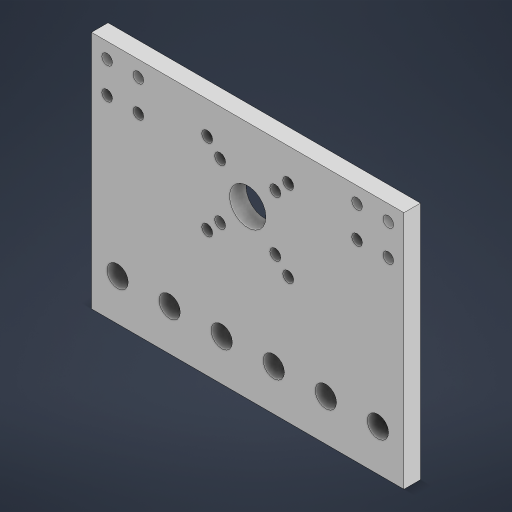
# Autodesk Inventor part: FirstStageMotorMountingPlate
Saved by Autodesk Inventor 2024 (Build 280153000, 153)
## iProperties
Created: 2024-01-05
Part Number: FirstStageMotorMountingPlate
Material: Generic
Document SubType Name: Modeling
Designer: avsar
Density: 1 g/cm^3
Appearance: Default
Author: avsar
Autodesk Inventor part; units mm, degrees
ref_plane "YZ Plane" through (0, 0, 0) normal (1, 0, 0) x (0, 1, 0)
ref_plane "XZ Plane" through (0, 0, 0) normal (0, 1, 0) x (-1, 0, 0)
ref_plane "XY Plane" through (0, 0, 0) normal (0, 0, 1) x (1, 0, 0)
sketch "Sketch1" plane through (0, 0, 0) normal (0, 0, 1) x (1, 0, 0)
  line L0 (-60, -46) -> (60, -46)
  line L1 (60, -46) -> (60, 46)
  line L2 (60, 46) -> (-60, 46)
  line L3 (-60, 46) -> (-60, -46)
  line L4 (-60, -46) -> (60, 46) construction
  line L5 (60, -46) -> (-60, 46) construction
  point P0 (0, 0)
  dimension "d0" = 120
  dimension "d1" = 92
  constraints: 12 end point, 2 midpoint, 2 parallel, 1 horizontal, 1 perpendicular
  measures "d0" distance of L2.end L1.end
  measures "d1" distance of L1.end L0.end
extrude "Extrusion1" add sketch "Sketch1" along normal mid plane 6.35
sketch "Sketch2" plane through (0, 0, 3.175) normal (0, 0, 1) x (1, 0, 0)
  circle A0 centre (0, 18) radius 7
  line L0 (-60, -46) -> (60, -46) projected
  circle A1 centre (-10.6066, 28.6066) radius 2.1
  line L1 (-10.6066, 28.6066) -> (0, 18) construction
  circle A2 centre (-15.5563, 33.5563) radius 2.1
  line L2 (-15.5563, 33.5563) -> (-10.6066, 28.6066) construction
  circle A3 centre (-15.5563, 2.4437) radius 2.1
  circle A4 centre (-10.6066, 7.3934) radius 2.1
  circle A5 centre (15.5563, 2.4437) radius 2.1
  circle A6 centre (10.6066, 7.3934) radius 2.1
  circle A7 centre (15.5563, 33.5563) radius 2.1
  circle A8 centre (10.6066, 28.6066) radius 2.1
  point P0 (0, 0)
  point P1 (0, -46)
  dimension "d4" = 14
  dimension "d6" = 64
  dimension "d7" = 4.2
  dimension "d8" = 45
  dimension "d9" = 15
  dimension "d10" = 4.2
  dimension "d11" = 7
  dimension "d14" = 360
  constraints: 9 centre point, 4 end point, 1 collinear, 1 midpoint, 1 vertical alignment, 17 other
  measures "d4" diameter of A0
  measures "d6" distance of point (0, -46) L1.end
  measures "d7" diameter of A1
  measures "d8" angle of L0 L1
  measures "d9" distance of L1.start L1.end
  measures "d10" diameter of A2
  measures "d11" distance of L2.start L1.start
extrude "Extrusion2" cut sketch "Sketch2" against normal through all
sketch "Sketch3" plane through (0, 0, 3.175) normal (0, 0, 1) x (1, 0, 0)
  circle A0 centre (-50, -30.125) radius 4.1
  line L0 (-60, -46) -> (60, -46) projected
  circle A1 centre (-30, -30.125) radius 4.1
  circle A2 centre (-10, -30.125) radius 4.1
  circle A3 centre (10, -30.125) radius 4.1
  circle A4 centre (30, -30.125) radius 4.1
  circle A5 centre (50, -30.125) radius 4.1
  point P0 (0, 0)
  point P1 (0, -46)
  dimension "d18" = 8.2
  dimension "d19" = 15.875
  dimension "d20" = 50
  dimension "d23" = 20
  constraints: 6 centre point, 1 horizontal, 1 midpoint, 10 other
  measures "d18" diameter of A0
  measures "d19" distance from line of L0 A0.centre
  measures "d20" horizontal distance of point (0, -46) A0.centre
  measures "d23" distance of A0.centre A1.centre
extrude "Extrusion3" cut sketch "Sketch3" against normal through all
sketch "Sketch4" plane through (0, 0, 3.175) normal (0, 0, 1) x (1, 0, 0)
  circle A0 centre (-48, 34) radius 2.5 construction
  circle A1 centre (-54, 40) radius 2.05
  circle A2 centre (-54, 28) radius 2.05
  circle A3 centre (-42, 28) radius 2.05
  circle A4 centre (-42, 40) radius 2.05
  line L0 (-60, 46) -> (-60, -46) projected
  line L1 (60, 46) -> (-60, 46) projected
  circle A5 centre (0, 18) radius 7 projected
  line L2 (0, 25) -> (0, 11) construction
  circle A6 centre (48, 34) radius 2.5 construction
  circle A7 centre (54, 40) radius 2.05
  circle A8 centre (54, 28) radius 2.05
  circle A9 centre (42, 28) radius 2.05
  circle A10 centre (42, 40) radius 2.05
  point P0 (0, 0)
  dimension "d30" = 5
  dimension "d31" = 4.1
  dimension "d32" = 6
  dimension "d33" = 6
  dimension "d36" = 360
  dimension "d38" = 12
  dimension "d39" = 12
  constraints: 10 centre point, 5 symmetric about line, 2 end point, 2 point on circle, 1 coincident, 1 midpoint, 1 vertical, 14 other
  measures "d30" diameter of A0
  measures "d31" diameter of A1
  measures "d32" horizontal distance of A1.centre A0.centre
  measures "d33" horizontal distance of A0.centre A1.centre
  measures "d38" distance from line of L0 A0.centre
  measures "d39" distance from line of L1 A0.centre
extrude "Extrusion4" cut sketch "Sketch4" against normal through all contours A1 | A2 | A3 | A4 | A7 | A8 | A9 | A10
body "Solid1"
